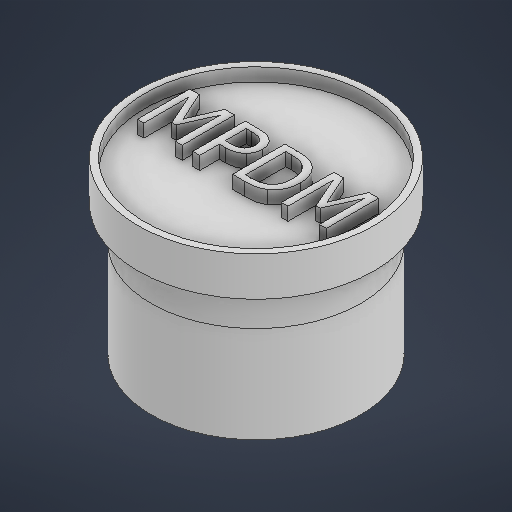
# Autodesk Inventor part: Pino
Saved by Autodesk Inventor 2026.1 (Build 301233020, 233B)
## iProperties
Created: 2025-11-10
Part Number: Pino
Material: Genérico
Document SubType Name: Modeling
Designer: luska
Density: 1 g/cm^3
Appearance: Padrão
Author: luska
Autodesk Inventor part; units mm, degrees
ref_plane "YZ Plane" through (0, 0, 0) normal (1, 0, 0) x (0, 1, 0)
ref_plane "XZ Plane" through (0, 0, 0) normal (0, 1, 0) x (-1, 0, 0)
ref_plane "XY Plane" through (0, 0, 0) normal (0, 0, 1) x (1, 0, 0)
sketch "Esboço1" plane through (0, 0, 0) normal (0, 1, 0) x (-1, 0, 0)
  circle A0 centre (0, 0) radius 4
  dimension "d0" = 8
  constraints: 1 centre point, 1 coincident
  measures "d0" diameter of A0
extrude "Extrusão1" add sketch "Esboço1" along normal blind 5
sketch "Esboço2" plane through (0, 0, 0) normal (0, -1, 0) x (1, 0, 0)
  circle A0 centre (0, 0) radius 3.1
  dimension "d3" = 6.2
  constraints: 1 centre point, 1 coincident
  measures "d3" diameter of A0
extrude "Extrusão2" cut sketch "Esboço2" against normal blind 3
sketch "Esboço3" plane through (0, 5, 0) normal (0, 1, 0) x (1, 0, 0)
  circle A0 centre (0, 0) radius 4.5
  dimension "d6" = 9
  constraints: 1 centre point, 1 coincident
  measures "d6" diameter of A0
extrude "Extrusão3" add sketch "Esboço3" along normal blind 1
fillet "Arredondamento1" radius 2 1 edges at (4, 5, 0)
sketch "Esboço4" plane through (0, 6, 0) normal (0, 1, 0) x (1, 0, 0)
  line L0 (-3.739, 1.0048) -> (0.0722, 1.0048) construction
  line L1 (0.0722, 1.0048) -> (0.0722, 0.0048) construction
  line L2 (0.0722, 0.0048) -> (-3.739, 0.0048) construction
  line L3 (-3.739, 0.0048) -> (-3.739, 1.0048) construction
  circle A0 centre (0, 0) radius 4.5
  circle A1 centre (0, 0) radius 4.25
  line L4 (-1.8216, -0.9952) -> (-2.0874, -0.9952)
  line L5 (-2.0874, -0.9952) -> (-2.0874, 0.7276)
  line L6 (-2.0874, 0.7276) -> (-2.6093, -0.4442)
  line L7 (-2.6093, -0.4442) -> (-2.7714, -0.4442)
  line L8 (-2.7714, -0.4442) -> (-3.2884, 0.7276)
  line L9 (-3.2884, 0.7276) -> (-3.2884, -0.9952)
  line L10 (-3.2884, -0.9952) -> (-3.5364, -0.9952)
  line L11 (-3.5364, -0.9952) -> (-3.5364, 1.0048)
  line L12 (-3.5364, 1.0048) -> (-3.1733, 1.0048)
  line L13 (-3.1733, 1.0048) -> (-2.6741, -0.1087)
  line L14 (-2.6741, -0.1087) -> (-2.1911, 1.0048)
  line L15 (-2.1911, 1.0048) -> (-1.8216, 1.0048)
  line L16 (-1.8216, 1.0048) -> (-1.8216, -0.9952)
  spline S0 degree 2 poles (-0.1522, 0.4018) (-0.1522, 0.2722) (-0.2446, 0.0388) (-0.3273, -0.0422) knots 0 0 0 1 2 2 2
  spline S1 degree 2 poles (-0.3273, -0.0422) (-0.431, -0.1444) (-0.7114, -0.2497) (-0.9253, -0.2497) knots 0 0 0 1 2 2 2
  line L17 (-0.9253, -0.2497) -> (-1.1506, -0.2497)
  line L18 (-1.1506, -0.2497) -> (-1.1506, -0.9952)
  line L19 (-1.1506, -0.9952) -> (-1.4164, -0.9952)
  line L20 (-1.4164, -0.9952) -> (-1.4164, 1.0048)
  line L21 (-1.4164, 1.0048) -> (-0.914, 1.0048)
  spline S2 degree 2 poles (-0.914, 1.0048) (-0.7357, 1.0048) (-0.4861, 0.9464) (-0.3905, 0.88) knots 0 0 0 1 2 2 2
  spline S3 degree 2 poles (-0.3905, 0.88) (-0.2787, 0.8038) (-0.1522, 0.5688) (-0.1522, 0.4018) knots 0 0 0 1 2 2 2
  spline S4 degree 2 poles (-0.4294, 0.3937) (-0.4294, 0.4975) (-0.5007, 0.6498) (-0.5736, 0.6984) knots 0 0 0 1 2 2 2
  spline S5 degree 2 poles (-0.5736, 0.6984) (-0.6369, 0.7406) (-0.8054, 0.7746) (-0.9302, 0.7746) knots 0 0 0 1 2 2 2
  line L22 (-0.9302, 0.7746) -> (-1.1506, 0.7746)
  line L23 (-1.1506, 0.7746) -> (-1.1506, -0.0228)
  line L24 (-1.1506, -0.0228) -> (-0.9691, -0.0228)
  spline S6 degree 2 poles (-0.9691, -0.0228) (-0.807, -0.0228) (-0.6077, 0.0291) (-0.5428, 0.0971) knots 0 0 0 1 2 2 2
  spline S7 degree 2 poles (-0.5428, 0.0971) (-0.4829, 0.1571) (-0.4294, 0.2981) (-0.4294, 0.3937) knots 0 0 0 1 2 2 2
  spline S8 degree 2 poles (1.6776, 0.0031) (1.6776, -0.2708) (1.4555, -0.7116) (1.2691, -0.8348) knots 0 0 0 1 2 2 2
  spline S9 degree 2 poles (1.2691, -0.8348) (1.1168, -0.9304) (0.804, -0.9952) (0.5609, -0.9952) knots 0 0 0 1 2 2 2
  line L25 (0.5609, -0.9952) -> (0.1006, -0.9952)
  line L26 (0.1006, -0.9952) -> (0.1006, 1.0048)
  line L27 (0.1006, 1.0048) -> (0.556, 1.0048)
  spline S10 degree 2 poles (0.556, 1.0048) (0.838, 1.0048) (1.1589, 0.9205) (1.2724, 0.8459) knots 0 0 0 1 2 2 2
  spline S11 degree 2 poles (1.2724, 0.8459) (1.4653, 0.7179) (1.6776, 0.2949) (1.6776, 0.0031) knots 0 0 0 1 2 2 2
  spline S12 degree 2 poles (1.4004, 0.0064) (1.4004, 0.2365) (1.2481, 0.5623) (1.0973, 0.6547) knots 0 0 0 1 2 2 2
  spline S13 degree 2 poles (1.0973, 0.6547) (0.9904, 0.7179) (0.7489, 0.7746) (0.569, 0.7746) knots 0 0 0 1 2 2 2
  line L28 (0.569, 0.7746) -> (0.3664, 0.7746)
  line L29 (0.3664, 0.7746) -> (0.3664, -0.7651)
  line L30 (0.3664, -0.7651) -> (0.569, -0.7651)
  spline S14 degree 2 poles (0.569, -0.7651) (0.7456, -0.7651) (1.0131, -0.7084) (1.1217, -0.6322) knots 0 0 0 1 2 2 2
  spline S15 degree 2 poles (1.1217, -0.6322) (1.261, -0.5382) (1.4004, -0.227) (1.4004, 0.0064) knots 0 0 0 1 2 2 2
  line L31 (3.6808, -0.9952) -> (3.415, -0.9952)
  line L32 (3.415, -0.9952) -> (3.415, 0.7276)
  line L33 (3.415, 0.7276) -> (2.8931, -0.4442)
  line L34 (2.8931, -0.4442) -> (2.7311, -0.4442)
  line L35 (2.7311, -0.4442) -> (2.214, 0.7276)
  line L36 (2.214, 0.7276) -> (2.214, -0.9952)
  line L37 (2.214, -0.9952) -> (1.9661, -0.9952)
  line L38 (1.9661, -0.9952) -> (1.9661, 1.0048)
  line L39 (1.9661, 1.0048) -> (2.3291, 1.0048)
  line L40 (2.3291, 1.0048) -> (2.8283, -0.1087)
  line L41 (2.8283, -0.1087) -> (3.3113, 1.0048)
  line L42 (3.3113, 1.0048) -> (3.6808, 1.0048)
  line L43 (3.6808, 1.0048) -> (3.6808, -0.9952)
  dimension "d2" = 0
  dimension "d10" = 9
  dimension "d11" = 8.5
  constraints: 2 centre point, 2 coincident, 2 other
  measures "d10" diameter of A0
  measures "d11" diameter of A1
extrude "Extrusão4" add sketch "Esboço4" along normal blind 0.5
